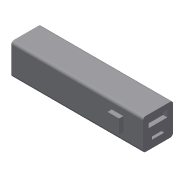
# Autodesk Inventor part: 00_Batterypack
Saved by Autodesk Inventor 2019.4 (Build 234330000, 330)
## iProperties
Created: 2021-06-03
Part Number: 00_Batterypack
Material: Generic
Document SubType Name: Modeling
Designer: diederichbenedict
Density: 1 g/cm^3
Appearance: Default
Author: diederichbenedict
Autodesk Inventor part; units mm, degrees
ref_plane "YZ Plane" through (0, 0, 0) normal (1, 0, 0) x (0, 1, 0)
ref_plane "XZ Plane" through (0, 0, 0) normal (0, 1, 0) x (-1, 0, 0)
ref_plane "XY Plane" through (0, 0, 0) normal (0, 0, 1) x (1, 0, 0)
sketch "Sketch1" plane through (0, 0, 0) normal (1, 0, 0) x (0, 1, 0)
  line L0 (-9.11, -10.73) -> (9.11, -10.73)
  line L1 (11.11, -8.73) -> (11.11, 8.73)
  line L2 (9.11, 10.73) -> (-9.11, 10.73)
  line L3 (-11.11, 8.73) -> (-11.11, -8.73)
  line L4 (-11.11, -10.73) -> (11.11, 10.73) construction
  line L5 (11.11, -10.73) -> (-11.11, 10.73) construction
  arc A0 (11.11, 8.73) -> (9.11, 10.73) centre (9.11, 8.73) ccw
  arc A1 (9.11, -10.73) -> (11.11, -8.73) centre (9.11, -8.73) ccw
  arc A2 (-11.11, -8.73) -> (-9.11, -10.73) centre (-9.11, -8.73) ccw
  arc A3 (-9.11, 10.73) -> (-11.11, 8.73) centre (-9.11, 8.73) ccw
  point P0 (0, 0)
  dimension "d0" = 22.22
  dimension "d1" = 21.46
  dimension "d2" = 2
  constraints: 12 end point, 8 point on circle, 8 point on line, 8 tangent, 4 centre point, 3 equal radius, 2 midpoint, 2 parallel, 1 horizontal, 1 perpendicular
  measures "d0" distance of L5.end L4.end
  measures "d1" distance of L4.end L5.start
  measures "d2" radius of A0
extrude "Extrusion1" add sketch "Sketch1" along normal blind 94
sketch "Sketch2" plane through (94, 0, 0) normal (1, 0, 0) x (0, 0, -1)
  line L0 (-6.6347, 7.2513) -> (6.6347, 7.2513)
  line L1 (6.6347, 7.2513) -> (6.6347, 2.4915)
  line L2 (6.6347, 2.4915) -> (-6.6347, 2.4915)
  line L3 (-6.6347, 2.4915) -> (-6.6347, 7.2513)
  line L4 (-6.6347, 7.2513) -> (6.6347, 2.4915) construction
  line L5 (6.6347, 7.2513) -> (-6.6347, 2.4915) construction
  line L6 (-4.3158, -3.8551) -> (4.3158, -3.8551)
  line L7 (4.3158, -3.8551) -> (4.3158, -5.8078)
  line L8 (4.3158, -5.8078) -> (-4.3158, -5.8078)
  line L9 (-4.3158, -5.8078) -> (-4.3158, -3.8551)
  line L10 (-4.3158, -3.8551) -> (4.3158, -5.8078) construction
  line L11 (4.3158, -3.8551) -> (-4.3158, -5.8078) construction
  point P0 (0, 0)
  point P1 (0, 4.8714)
  point P2 (0, -4.8314)
  constraints: 24 end point, 4 midpoint, 4 parallel, 2 horizontal, 2 perpendicular
extrude "Extrusion2" cut sketch "Sketch2" against normal blind 3
sketch "Sketch3" plane through (0, -9.11, 10.73) normal (0, 0, 1) x (1, 0, 0)
  line L0 (0, 18.22) -> (0, 0) projected
  line L1 (0, 0) -> (94, 0) projected
  line L2 (94, 18.22) -> (94, 0) projected
  line L3 (0, 18.22) -> (94, 18.22) projected
  line L4 (71.8, 14.11) -> (80, 14.11)
  line L5 (80, 14.11) -> (80, 4.11)
  line L6 (80, 4.11) -> (71.8, 4.11)
  line L7 (71.8, 4.11) -> (71.8, 14.11)
  line L8 (71.8, 14.11) -> (80, 4.11) construction
  line L9 (80, 14.11) -> (71.8, 4.11) construction
  point P0 (0, 9.11)
  point P1 (75.9, 9.11)
  dimension "d7" = 8.2
  dimension "d8" = 10
  dimension "d9" = 14
  constraints: 12 end point, 2 midpoint, 2 parallel, 1 horizontal, 1 perpendicular
  measures "d7" distance of L5.end L6.end
  measures "d8" distance of L4.end L5.end
  measures "d9" distance between parallel lines of L5 L2
extrude "Extrusion3" add sketch "Sketch3" along normal blind 3 contours L4 L5 L6 L7
body "Solid1"
